Autodesk Inventor part; units mm, degrees
(part 2 of 2)
  spline S331 degree 2 poles (167.9994, 31.495) (169.0908, 32.2557) (170.7003, 32.3439) knots 0 0 0 1 1 1
  line L176 (170.2153, 20.1951) -> (170.2153, 19.1368)
  spline S332 degree 2 poles (170.2153, 19.1368) (169.4546, 19.1368) (168.5286, 19.5667) knots 0 0 0 1 1 1
  spline S333 degree 2 poles (168.5286, 19.5667) (168.1868, 19.7321) (167.9222, 19.8203) (167.801, 19.8203) knots 0 0 0 1 2 2 2
  spline S334 degree 2 poles (167.801, 19.8203) (167.6246, 19.8203) (167.4372, 19.699) (167.2277, 19.4565) knots 0 0 0 1 2 2 2
  spline S335 degree 2 poles (167.2277, 19.4565) (167.0623, 19.2581) (166.8639, 19.2581) knots 0 0 0 1 1 1
  spline S336 degree 2 poles (166.8639, 19.2581) (166.3457, 19.2581) (166.3457, 20.0628) knots 0 0 0 1 1 1
  line L177 (166.3457, 20.0628) -> (166.3457, 23.4473)
  spline S337 degree 2 poles (166.3457, 23.4473) (166.3457, 23.7009) (166.6434, 24.0647) (166.8639, 24.0757) knots 0 0 0 1 2 2 2
  spline S338 degree 2 poles (166.8639, 24.0757) (167.0733, 24.0867) (167.3049, 23.8331) (167.3931, 23.5134) knots 0 0 0 1 2 2 2
  spline S339 degree 2 poles (167.3931, 23.5134) (167.6025, 22.7197) (168.4073, 21.3196) (168.9475, 20.8456) knots 0 0 0 1 2 2 2
  spline S340 degree 2 poles (168.9475, 20.8456) (169.4987, 20.3384) (170.2153, 20.1951) knots 0 0 0 1 1 1
  line L178 (171.439, 31.2745) -> (171.439, 32.2998)
  spline S341 degree 2 poles (171.439, 32.2998) (172.0012, 32.2557) (172.817, 32.0352) (173.5667, 31.7155) knots 0 0 0 1 2 2 2
  spline S342 degree 2 poles (173.5667, 31.7155) (173.7541, 31.6384) (173.8753, 31.6384) knots 0 0 0 1 1 1
  spline S343 degree 2 poles (173.8753, 31.6384) (174.0517, 31.6384) (174.1399, 31.7596) knots 0 0 0 1 1 1
  line L179 (174.1399, 31.7596) -> (174.3384, 32.0352)
  spline S344 degree 2 poles (174.3384, 32.0352) (174.4927, 32.2447) (174.7022, 32.2447) knots 0 0 0 1 1 1
  spline S345 degree 2 poles (174.7022, 32.2447) (174.9557, 32.2447) (175.1872, 31.8809) (175.1872, 31.495) knots 0 0 0 1 2 2 2
  line L180 (175.1872, 31.495) -> (175.1872, 28.4193)
  spline S346 degree 2 poles (175.1872, 28.4193) (175.1872, 28.1436) (174.8786, 27.8019) (174.636, 27.8019) knots 0 0 0 1 2 2 2
  spline S347 degree 2 poles (174.636, 27.8019) (174.4486, 27.8019) (174.2943, 27.9232) knots 0 0 0 1 1 1
  spline S348 degree 2 poles (174.2943, 27.9232) (174.2061, 28.0003) (174.1069, 28.2098) (174.0628, 28.4634) knots 0 0 0 1 2 2 2
  spline S349 degree 2 poles (174.0628, 28.4634) (173.9635, 28.9264) (173.4564, 29.8855) (173.1257, 30.2713) knots 0 0 0 1 2 2 2
  spline S350 degree 2 poles (173.1257, 30.2713) (172.4532, 31.032) (171.439, 31.2745) knots 0 0 0 1 1 1
  line L181 (182.1656, 32.0903) -> (182.1656, 19.3903)
  line L182 (182.1656, 19.3903) -> (178.0205, 19.3903)
  line L183 (178.0205, 19.3903) -> (177.7779, 19.3903)
  spline S351 degree 2 poles (177.7779, 19.3903) (177.4472, 19.3903) (177.0834, 19.6439) (177.0834, 19.8754) knots 0 0 0 1 2 2 2
  spline S352 degree 2 poles (177.0834, 19.8754) (177.0834, 20.2502) (177.4582, 20.3715) knots 0 0 0 1 1 1
  spline S353 degree 2 poles (177.4582, 20.3715) (177.7669, 20.4818) (177.8661, 20.5259) (177.9213, 20.614) knots 0 0 0 1 2 2 2
  spline S354 degree 2 poles (177.9213, 20.614) (178.0315, 20.7574) (178.0315, 21.0881) knots 0 0 0 1 1 1
  line L184 (178.0315, 21.0881) -> (178.0315, 30.3926)
  spline S355 degree 2 poles (178.0315, 30.3926) (178.0315, 30.7233) (177.9213, 30.8667) knots 0 0 0 1 1 1
  spline S356 degree 2 poles (177.9213, 30.8667) (177.8661, 30.9548) (177.7669, 30.9989) (177.4582, 31.0982) knots 0 0 0 1 2 2 2
  spline S357 degree 2 poles (177.4582, 31.0982) (177.0834, 31.2194) (177.0834, 31.6053) knots 0 0 0 1 1 1
  spline S358 degree 2 poles (177.0834, 31.6053) (177.0834, 31.8368) (177.4472, 32.0903) (177.7779, 32.0903) knots 0 0 0 1 2 2 2
  line L185 (177.7779, 32.0903) -> (178.0205, 32.0903)
  line L186 (178.0205, 32.0903) -> (182.1656, 32.0903)
  line L187 (183.0035, 19.3903) -> (183.0035, 20.3936)
  spline S359 degree 2 poles (183.0035, 20.3936) (183.6098, 20.4818) (184.4036, 20.8235) (184.8004, 21.1653) knots 0 0 0 1 2 2 2
  spline S360 degree 2 poles (184.8004, 21.1653) (185.1973, 21.507) (185.6714, 22.2456) (185.8918, 22.852) knots 0 0 0 1 2 2 2
  spline S361 degree 2 poles (185.8918, 22.852) (185.9911, 23.1496) (186.2115, 23.3591) (186.41, 23.3591) knots 0 0 0 1 2 2 2
  spline S362 degree 2 poles (186.41, 23.3591) (186.6635, 23.3591) (186.873, 23.0504) (186.873, 22.6756) knots 0 0 0 1 2 2 2
  line L188 (186.873, 22.6756) -> (186.873, 19.3903)
  line L189 (186.873, 19.3903) -> (183.0035, 19.3903)
  line L190 (182.9924, 32.0903) -> (186.7407, 32.0903)
  line L191 (186.7407, 32.0903) -> (186.7407, 28.7941)
  spline S363 degree 2 poles (186.7407, 28.7941) (186.7407, 28.5074) (186.5202, 28.2539) (186.2777, 28.2539) knots 0 0 0 1 2 2 2
  spline S364 degree 2 poles (186.2777, 28.2539) (186.0682, 28.2539) (185.8808, 28.4193) (185.8036, 28.6838) knots 0 0 0 1 2 2 2
  spline S365 degree 2 poles (185.8036, 28.6838) (185.4509, 29.7532) (184.0839, 30.8887) (182.9924, 30.9989) knots 0 0 0 1 2 2 2
  line L192 (182.9924, 30.9989) -> (182.9924, 32.0903)
  line L193 (182.9483, 25.3104) -> (182.9483, 26.3908)
  spline S366 degree 2 poles (182.9483, 26.3908) (183.4885, 26.6554) (184.0067, 27.2727) (184.1279, 27.7798) knots 0 0 0 1 2 2 2
  spline S367 degree 2 poles (184.1279, 27.7798) (184.2051, 28.1326) (184.4477, 28.4082) (184.6681, 28.4082) knots 0 0 0 1 2 2 2
  spline S368 degree 2 poles (184.6681, 28.4082) (184.9658, 28.4082) (185.076, 28.1767) knots 0 0 0 1 1 1
  spline S369 degree 2 poles (185.076, 28.1767) (185.1422, 28.0555) (185.1422, 27.6255) knots 0 0 0 1 1 1
  line L194 (185.1422, 27.6255) -> (185.1422, 24.0757)
  spline S370 degree 2 poles (185.1422, 24.0757) (185.1422, 23.6347) (184.9437, 23.304) (184.6902, 23.304) knots 0 0 0 1 2 2 2
  spline S371 degree 2 poles (184.6902, 23.304) (184.4697, 23.304) (184.2272, 23.5686) (184.161, 23.8772) knots 0 0 0 1 2 2 2
  spline S372 degree 2 poles (184.161, 23.8772) (183.9957, 24.5167) (183.4114, 25.2002) (182.9483, 25.3104) knots 0 0 0 1 2 2 2
  line L195 (198.68, 31.3407) -> (198.68, 32.3439)
  spline S373 degree 2 poles (198.68, 32.3439) (199.6832, 32.2998) (201.3479, 31.5722) (202.0645, 30.8667) knots 0 0 0 1 2 2 2
  spline S374 degree 2 poles (202.0645, 30.8667) (203.9607, 29.0146) (203.9607, 25.7293) knots 0 0 0 1 1 1
  spline S375 degree 2 poles (203.9607, 25.7293) (203.9607, 22.4992) (202.1527, 20.6912) knots 0 0 0 1 1 1
  spline S376 degree 2 poles (202.1527, 20.6912) (200.7526, 19.3022) (198.68, 19.1368) knots 0 0 0 1 1 1
  line L196 (198.68, 19.1368) -> (198.68, 20.162)
  spline S377 degree 2 poles (198.68, 20.162) (198.9226, 20.2172) (199.1871, 20.3936) (199.2974, 20.5589) knots 0 0 0 1 2 2 2
  spline S378 degree 2 poles (199.2974, 20.5589) (199.551, 20.9448) (199.551, 21.7165) knots 0 0 0 1 1 1
  line L197 (199.551, 21.7165) -> (199.551, 30.0288)
  spline S379 degree 2 poles (199.551, 30.0288) (199.551, 30.5249) (199.3856, 30.8115) knots 0 0 0 1 1 1
  spline S380 degree 2 poles (199.3856, 30.8115) (199.2753, 31.01) (198.9667, 31.2305) (198.68, 31.3407) knots 0 0 0 1 2 2 2
  spline S381 degree 2 poles (197.9194, 31.3407) (197.4453, 31.1643) (197.0595, 30.591) (197.0595, 30.0288) knots 0 0 0 1 2 2 2
  line L198 (197.0595, 30.0288) -> (197.0595, 21.7165)
  spline S382 degree 2 poles (197.0595, 21.7165) (197.0595, 20.9007) (197.2799, 20.5589) knots 0 0 0 1 1 1
  spline S383 degree 2 poles (197.2799, 20.5589) (197.4563, 20.2833) (197.9194, 20.162) knots 0 0 0 1 1 1
  line L199 (197.9194, 20.162) -> (197.9194, 19.1368)
  spline S384 degree 2 poles (197.9194, 19.1368) (195.8578, 19.3022) (194.4577, 20.6912) knots 0 0 0 1 1 1
  spline S385 degree 2 poles (194.4577, 20.6912) (192.6497, 22.4992) (192.6497, 25.7293) knots 0 0 0 1 1 1
  spline S386 degree 2 poles (192.6497, 25.7293) (192.6497, 27.3499) (193.6089, 29.9627) (194.5459, 30.8667) knots 0 0 0 1 2 2 2
  spline S387 degree 2 poles (194.5459, 30.8667) (195.2625, 31.5722) (196.9161, 32.2998) (197.9194, 32.3439) knots 0 0 0 1 2 2 2
  line L200 (197.9194, 32.3439) -> (197.9194, 31.3407)
  line L201 (210.3768, 32.0903) -> (215.3267, 23.4914)
  line L202 (215.3267, 23.4914) -> (215.3267, 19.3903)
  line L203 (215.3267, 19.3903) -> (212.7911, 19.3903)
  line L204 (212.7911, 19.3903) -> (206.4742, 30.2713)
  spline S388 degree 2 poles (206.4742, 30.2713) (206.2648, 30.6351) (206.0002, 30.9107) (205.8017, 30.9769) knots 0 0 0 1 2 2 2
  line L205 (205.8017, 30.9769) -> (205.449, 31.1092)
  spline S389 degree 2 poles (205.449, 31.1092) (205.3056, 31.1533) (205.1403, 31.3958) (205.1403, 31.5391) knots 0 0 0 1 2 2 2
  spline S390 degree 2 poles (205.1403, 31.5391) (205.1403, 31.7045) (205.3056, 31.9691) (205.449, 32.0242) knots 0 0 0 1 2 2 2
  spline S391 degree 2 poles (205.449, 32.0242) (205.6033, 32.0903) (206.3089, 32.0903) knots 0 0 0 1 1 1
  line L206 (206.3089, 32.0903) -> (210.3768, 32.0903)
  line L207 (206.4742, 28.8161) -> (207.4554, 27.1845)
  line L208 (207.4554, 27.1845) -> (207.4554, 22.2015)
  spline S392 degree 2 poles (207.4554, 22.2015) (207.4554, 21.5511) (207.8964, 20.7133) (208.3704, 20.4377) knots 0 0 0 1 2 2 2
  line L209 (208.3704, 20.4377) -> (208.646, 20.2833)
  spline S393 degree 2 poles (208.646, 20.2833) (208.8885, 20.14) (208.8885, 19.8644) knots 0 0 0 1 1 1
  spline S394 degree 2 poles (208.8885, 19.8644) (208.8885, 19.6549) (208.7121, 19.5116) knots 0 0 0 1 1 1
  spline S395 degree 2 poles (208.7121, 19.5116) (208.5578, 19.3903) (208.0948, 19.3903) knots 0 0 0 1 1 1
  line L210 (208.0948, 19.3903) -> (205.9561, 19.3903)
  spline S396 degree 2 poles (205.9561, 19.3903) (205.1072, 19.3903) (205.1072, 19.8754) knots 0 0 0 1 1 1
  spline S397 degree 2 poles (205.1072, 19.8754) (205.1072, 20.0408) (205.2836, 20.2392) (205.5812, 20.4046) knots 0 0 0 1 2 2 2
  spline S398 degree 2 poles (205.5812, 20.4046) (206.4742, 20.9007) (206.4742, 22.2015) knots 0 0 0 1 1 1
  line L211 (206.4742, 22.2015) -> (206.4742, 28.8161)
  line L212 (215.3267, 24.9797) -> (214.3456, 26.6443)
  line L213 (214.3456, 26.6443) -> (214.3456, 29.224)
  spline S399 degree 2 poles (214.3456, 29.224) (214.3456, 30.0068) (213.8936, 30.8336) (213.3093, 31.1312) knots 0 0 0 1 2 2 2
  spline S400 degree 2 poles (213.3093, 31.1312) (213.1219, 31.2194) (212.9675, 31.4399) (212.9675, 31.6053) knots 0 0 0 1 2 2 2
  spline S401 degree 2 poles (212.9675, 31.6053) (212.9675, 31.8588) (213.2983, 32.0903) (213.6621, 32.0903) knots 0 0 0 1 2 2 2
  line L214 (213.6621, 32.0903) -> (215.9772, 32.0903)
  spline S402 degree 2 poles (215.9772, 32.0903) (216.4512, 32.0903) (216.6056, 31.936) knots 0 0 0 1 1 1
  spline S403 degree 2 poles (216.6056, 31.936) (216.7599, 31.7927) (216.7599, 31.5832) knots 0 0 0 1 1 1
  spline S404 degree 2 poles (216.7599, 31.5832) (216.7599, 31.3958) (216.5835, 31.1974) (216.2528, 31.032) knots 0 0 0 1 2 2 2
  spline S405 degree 2 poles (216.2528, 31.032) (215.7567, 30.7785) (215.5031, 30.2603) knots 0 0 0 1 1 1
  spline S406 degree 2 poles (215.5031, 30.2603) (215.3267, 29.8745) (215.3267, 29.224) knots 0 0 0 1 1 1
  line L215 (215.3267, 29.224) -> (215.3267, 24.9797)
  line L216 (222.9776, 19.3903) -> (218.8325, 19.3903)
  line L217 (218.8325, 19.3903) -> (218.5899, 19.3903)
  spline S407 degree 2 poles (218.5899, 19.3903) (218.2592, 19.3903) (217.8954, 19.6439) (217.8954, 19.8754) knots 0 0 0 1 2 2 2
  spline S408 degree 2 poles (217.8954, 19.8754) (217.8954, 20.2502) (218.2702, 20.3715) knots 0 0 0 1 1 1
  spline S409 degree 2 poles (218.2702, 20.3715) (218.5789, 20.4818) (218.6781, 20.5259) (218.7332, 20.614) knots 0 0 0 1 2 2 2
  spline S410 degree 2 poles (218.7332, 20.614) (218.8435, 20.7574) (218.8435, 21.0881) knots 0 0 0 1 1 1
  line L218 (218.8435, 21.0881) -> (218.8435, 30.3926)
  spline S411 degree 2 poles (218.8435, 30.3926) (218.8435, 30.7233) (218.7332, 30.8667) knots 0 0 0 1 1 1
  spline S412 degree 2 poles (218.7332, 30.8667) (218.6781, 30.9548) (218.5789, 30.9989) (218.2702, 31.0982) knots 0 0 0 1 2 2 2
  spline S413 degree 2 poles (218.2702, 31.0982) (217.8954, 31.2194) (217.8954, 31.6053) knots 0 0 0 1 1 1
  spline S414 degree 2 poles (217.8954, 31.6053) (217.8954, 31.8368) (218.2592, 32.0903) (218.5899, 32.0903) knots 0 0 0 1 2 2 2
  line L219 (218.5899, 32.0903) -> (218.8325, 32.0903)
  line L220 (218.8325, 32.0903) -> (222.9886, 32.0903)
  line L221 (222.9886, 32.0903) -> (223.3083, 32.0903)
  spline S415 degree 2 poles (223.3083, 32.0903) (223.7162, 32.0903) (223.8926, 31.9801) knots 0 0 0 1 1 1
  spline S416 degree 2 poles (223.8926, 31.9801) (224.1352, 31.8258) (224.1352, 31.5832) knots 0 0 0 1 1 1
  spline S417 degree 2 poles (224.1352, 31.5832) (224.1352, 31.1753) (223.6832, 31.0761) knots 0 0 0 1 1 1
  spline S418 degree 2 poles (223.6832, 31.0761) (223.3194, 30.9879) (223.1871, 30.9328) (223.1209, 30.8556) knots 0 0 0 1 2 2 2
  spline S419 degree 2 poles (223.1209, 30.8556) (222.9776, 30.6792) (222.9776, 30.3265) knots 0 0 0 1 1 1
  line L222 (222.9776, 30.3265) -> (222.9776, 19.3903)
  line L223 (223.7383, 19.3903) -> (223.7383, 20.4377)
  spline S420 degree 2 poles (223.7383, 20.4377) (224.1903, 20.5148) (224.7194, 20.7243) (224.962, 20.9117) knots 0 0 0 1 2 2 2
  spline S421 degree 2 poles (224.962, 20.9117) (225.3589, 21.2204) (226.0093, 22.3008) (226.2077, 22.9622) knots 0 0 0 1 2 2 2
  spline S422 degree 2 poles (226.2077, 22.9622) (226.3621, 23.4693) (226.6046, 23.8001) (226.8471, 23.8001) knots 0 0 0 1 2 2 2
  spline S423 degree 2 poles (226.8471, 23.8001) (227.1117, 23.8001) (227.233, 23.5906) knots 0 0 0 1 1 1
  spline S424 degree 2 poles (227.233, 23.5906) (227.2881, 23.4804) (227.2881, 23.1717) knots 0 0 0 1 1 1
  line L224 (227.2881, 23.1717) -> (227.2881, 19.3903)
  line L225 (227.2881, 19.3903) -> (223.7383, 19.3903)
  line L226 (234.9279, 25.2112) -> (234.9279, 21.1542)
  spline S425 degree 2 poles (234.9279, 21.1542) (234.9279, 20.7904) (235.0713, 20.6361) knots 0 0 0 1 1 1
  spline S426 degree 2 poles (235.0713, 20.6361) (235.1374, 20.5479) (235.2697, 20.4928) (235.6335, 20.4046) knots 0 0 0 1 2 2 2
  spline S427 degree 2 poles (235.6335, 20.4046) (236.0855, 20.3054) (236.0855, 19.8975) knots 0 0 0 1 1 1
  spline S428 degree 2 poles (236.0855, 19.8975) (236.0855, 19.6219) (235.8319, 19.4785) knots 0 0 0 1 1 1
  spline S429 degree 2 poles (235.8319, 19.4785) (235.6886, 19.3903) (235.2587, 19.3903) knots 0 0 0 1 1 1
  line L227 (235.2587, 19.3903) -> (234.939, 19.3903)
  line L228 (234.939, 19.3903) -> (230.7828, 19.3903)
  line L229 (230.7828, 19.3903) -> (230.4741, 19.3903)
  spline S430 degree 2 poles (230.4741, 19.3903) (230.0552, 19.3903) (229.8898, 19.5006) knots 0 0 0 1 1 1
  spline S431 degree 2 poles (229.8898, 19.5006) (229.6473, 19.6549) (229.6473, 19.8975) knots 0 0 0 1 1 1
  spline S432 degree 2 poles (229.6473, 19.8975) (229.6473, 20.3054) (230.0993, 20.4046) knots 0 0 0 1 1 1
  spline S433 degree 2 poles (230.0993, 20.4046) (230.4631, 20.4928) (230.5844, 20.5479) (230.6505, 20.6361) knots 0 0 0 1 2 2 2
  spline S434 degree 2 poles (230.6505, 20.6361) (230.7938, 20.7904) (230.7938, 21.1542) knots 0 0 0 1 1 1
  line L230 (230.7938, 21.1542) -> (230.7938, 24.2962)
  line L231 (230.7938, 24.2962) -> (228.159, 30.58)
  spline S435 degree 2 poles (228.159, 30.58) (228.0157, 30.9328) (227.7401, 31.0982) knots 0 0 0 1 1 1
  spline S436 degree 2 poles (227.7401, 31.0982) (227.4976, 31.2525) (227.3542, 31.4399) (227.3542, 31.6053) knots 0 0 0 1 2 2 2
  spline S437 degree 2 poles (227.3542, 31.6053) (227.3542, 32.0903) (228.0598, 32.0903) knots 0 0 0 1 1 1
  line L232 (228.0598, 32.0903) -> (232.6239, 32.0903)
  spline S438 degree 2 poles (232.6239, 32.0903) (232.9766, 32.0903) (233.12, 32.0022) knots 0 0 0 1 1 1
  spline S439 degree 2 poles (233.12, 32.0022) (233.3515, 31.8588) (233.3515, 31.6163) knots 0 0 0 1 1 1
  spline S440 degree 2 poles (233.3515, 31.6163) (233.3515, 31.3186) (233.0869, 31.1533) knots 0 0 0 1 1 1
  line L233 (233.0869, 31.1533) -> (232.8113, 30.9879)
  spline S441 degree 2 poles (232.8113, 30.9879) (232.6569, 30.8777) (232.6569, 30.6792) knots 0 0 0 1 1 1
  spline S442 degree 2 poles (232.6569, 30.6792) (232.6569, 30.4477) (232.7562, 30.2162) knots 0 0 0 1 1 1
  line L234 (232.7562, 30.2162) -> (234.9279, 25.2112)
  line L235 (235.2917, 26.0931) -> (234.7626, 27.3168)
  line L236 (234.7626, 27.3168) -> (235.7437, 29.4996)
  spline S443 degree 2 poles (235.7437, 29.4996) (235.865, 29.7863) (235.865, 30.2603) knots 0 0 0 1 1 1
  spline S444 degree 2 poles (235.865, 30.2603) (235.865, 30.8005) (235.2697, 31.043) knots 0 0 0 1 1 1
  spline S445 degree 2 poles (235.2697, 31.043) (234.95, 31.1643) (234.7516, 31.3627) (234.7516, 31.5722) knots 0 0 0 1 2 2 2
  spline S446 degree 2 poles (234.7516, 31.5722) (234.7516, 31.8258) (234.9169, 31.947) knots 0 0 0 1 1 1
  spline S447 degree 2 poles (234.9169, 31.947) (235.0272, 32.0352) (235.3028, 32.0903) (235.6556, 32.0903) knots 0 0 0 1 2 2 2
  line L237 (235.6556, 32.0903) -> (237.9486, 32.0903)
  spline S448 degree 2 poles (237.9486, 32.0903) (238.599, 32.0903) (238.599, 31.5722) knots 0 0 0 1 1 1
  spline S449 degree 2 poles (238.599, 31.5722) (238.599, 31.3848) (238.4227, 31.1753) (238.1691, 31.0651) knots 0 0 0 1 2 2 2
  spline S450 degree 2 poles (238.1691, 31.0651) (237.7171, 30.8667) (237.5187, 30.6572) knots 0 0 0 1 1 1
  spline S451 degree 2 poles (237.5187, 30.6572) (237.2431, 30.3595) (237.0556, 29.9737) knots 0 0 0 1 1 1
  line L238 (237.0556, 29.9737) -> (236.8462, 29.4996)
  line L239 (236.8462, 29.4996) -> (235.2917, 26.0931)
  point P0 (0, 0)
  constraints: 4 point on line, 4 other
extrude "Extrusion2" cut sketch "Sketch2" against normal blind 25.4
body "Solid1"
